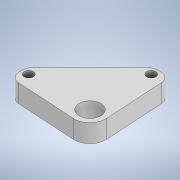
# Autodesk Inventor part: bell_crank_v1
Saved by Autodesk Inventor 2022 (Build 260153000, 153)
## iProperties
Created: 2022-05-22
Part Number: bell_crank_v1
Material: Generic
Document SubType Name: Modeling
Designer: kylem
Density: 1 g/cm^3
Appearance: Default
Author: kylem
Autodesk Inventor part; units mm, degrees
ref_plane "YZ Plane" through (0, 0, 0) normal (1, 0, 0) x (0, 1, 0)
ref_plane "XZ Plane" through (0, 0, 0) normal (0, 1, 0) x (-1, 0, 0)
ref_plane "XY Plane" through (0, 0, 0) normal (0, 0, 1) x (1, 0, 0)
sketch "Sketch1" plane through (0, 0, 0) normal (0, 1, 0) x (-1, 0, 0)
  circle A0 centre (0, 0) radius 15
  line L0 (0, 0) -> (14.7721, 2.6047)
  line L1 (0, 0) -> (15, 0) construction
  line L2 (0, 0) -> (-2.6047, -14.7721)
  line L3 (0, 0) -> (15, 0) construction
  line L4 (15, 0) -> (13.5, 0)
  circle A1 centre (13.5, 0) radius 1
  line L5 (0, -15) -> (0, -13.5)
  circle A2 centre (0, -13.5) radius 1
  dimension "d0" = 30
  dimension "d1" = 10
  dimension "d2" = 100
  dimension "d3" = 1.5
  dimension "d4" = 2
  dimension "d5" = 1.5
  dimension "d6" = 2
  constraints: 12 end point, 3 centre point, 3 coincident, 3 point on circle, 2 equal length, 2 horizontal, 1 point on line, 1 vertical
  measures "d0" diameter of A0
  measures "d1" angle of L1 L0
  measures "d2" angle of L2 L3
  measures "d3" distance of L3.end L4.end
  measures "d4" diameter of A1
  measures "d5" distance of L5.start L5.end
  measures "d6" diameter of A2
extrude "Extrusion1" add sketch "Sketch1" along normal blind 4 contours A0 L2 L0 picked at (8.114, -3.2724)
sketch "Sketch2" plane through (0, 4, 0) normal (0, 1, 0) x (1, 0, 0)
  line L0 (0, 0) -> (2.6047, 14.7721) projected
  circle A0 centre (0, 0) radius 1
  dimension "d9" = 2
  constraints: 1 centre point, 1 coincident
  measures "d9" diameter of A0
extrude "Extrusion2" cut sketch "Sketch2" against normal blind 4
sketch "Sketch3" plane through (0, 4, 0) normal (0, 1, 0) x (1, 0, 0)
  circle A0 centre (0, 0) radius 2.375
  dimension "d12" = 4.75
  constraints: 1 centre point, 1 coincident
  measures "d12" diameter of A0
extrude "Extrusion3" cut sketch "Sketch3" against normal blind 10
sketch "Sketch4" plane through (0, 4, 0) normal (0, 1, 0) x (1, 0, 0)
  circle A0 centre (0, 0) radius 3.5
  line L0 (0.4124, 2.3389) -> (2.6047, 14.7721) projected
  circle A1 centre (0, 0) radius 2.375
  dimension "d15" = 7
  constraints: 2 coincident, 1 centre point, 3 other
  measures "d15" diameter of A0
extrude "Extrusion4" add sketch "Sketch4" against normal blind 4
sketch "Sketch5" plane through (0, 4, 0) normal (0, 1, 0) x (1, 0, 0)
  arc A0 (2.6047, 14.7721) -> (-14.7721, -2.6047) centre (0, 0) ccw projected
  line L0 (2.6047, 14.7721) -> (3.4935, 0.2133)
  arc A1 (-3.4468, -0.6078) -> (0.6078, 3.4468) centre (0, 0) ccw projected
  line L1 (-14.7721, -2.6047) -> (-3.4468, -0.6078) projected
  line L2 (-14.7721, -2.6047) -> (-0.2133, -3.4935)
  line L3 (-14.7721, -2.6047) -> (-3.4468, -0.6078)
  line L4 (0.6078, 3.4468) -> (2.6047, 14.7721) projected
  line L5 (2.6047, 14.7721) -> (0.6078, 3.4468)
  circle A2 centre (0, 0) radius 3.5
  constraints: 8 end point, 2 point on circle, 2 tangent, 1 coincident, 1 collinear, 3 other
extrude "Extrusion5" add sketch "Sketch5" against normal blind 4 contours L0 A1 L4 | L1 A1 L2
fillet "Fillet1" radius 2 2 edges at (-14.7721, 2, 2.6047) (2.6047, 2, -14.7721)
sketch "Sketch6" plane through (0, 4, 0) normal (0, 1, 0) x (1, 0, 0)
  circle A0 centre (0, 13.5) radius 1 projected
  line L0 (-1, 13.5) -> (-1, 18.6359)
  circle A1 centre (-13.5, 0) radius 1 projected
  line L1 (-13.5, 1) -> (-18.0154, 1)
  arc A2 (0.8197, 14.9776) -> (-14.9776, -0.8197) centre (0, 0) ccw projected
  line L2 (-14.9666, 1) -> (-1, 14.9666)
  line L3 (-1, 14.9666) -> (-5.2156, 17.9633)
  line L4 (-5.2156, 17.9633) -> (-18.2143, 2.956)
  line L5 (-18.2143, 2.956) -> (-14.9666, 1)
  constraints: 12 end point, 2 horizontal, 2 point on circle, 2 point on line, 2 vertical, 1 horizontal alignment, 1 vertical alignment, 2 other
extrude "Extrusion6" cut sketch "Sketch6" against normal blind 40 contours L2 A2
fillet "Fillet2" radius 2 2 edges at (-1, 2, -14.9666) (-14.9666, 2, -1)
body "Solid1"
